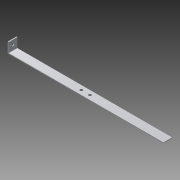
# Autodesk Inventor part: 爪２
Saved by Autodesk Inventor 2015 (Build 190159000, 159)
## iProperties
Created: 2015-05-17
Part Number: 爪２
Material: アルミニウム 6061
Document SubType Name: Modeling
Designer: Shun
Density: 2.7 g/cm^3
Appearance: アルミニウム - フラット
Mass: 5.09186 g
Surface Area: 42.039 cm^2
Volume: 1.88587 cm^3
Author: Shun
Autodesk Inventor part; units mm, degrees
ref_plane "YZ Plane" through (0, 0, 0) normal (1, 0, 0) x (0, 1, 0)
ref_plane "XZ Plane" through (0, 0, 0) normal (0, 1, 0) x (-1, 0, 0)
ref_plane "XY Plane" through (0, 0, 0) normal (0, 0, 1) x (1, 0, 0)
sketch "スケッチ1" plane through (0, 0, 0) normal (0, 0, 1) x (1, 0, 0)
  line L0 (-17.6, 4.0667) -> (162.4, 4.0667)
  line L1 (162.4, 4.0667) -> (162.4, -5.9333)
  line L2 (162.4, -5.9333) -> (-17.6, -5.9333)
  line L3 (-17.6, -5.9333) -> (-17.6, 4.0667)
  point P0 (0, 0)
  dimension "d0" = 10
  dimension "d1" = 180
  constraints: 8 end point, 2 parallel, 1 horizontal, 1 perpendicular
  measures "d0" distance of L2.end L0.start
  measures "d1" distance of L0.start L0.end
extrude "押し出し1" add sketch "スケッチ1" along normal blind 1
sketch "スケッチ3" plane through (0, 0, 1) normal (0, 0, 1) x (1, 0, 0)
  circle A0 centre (62.4, -0.9333) radius 1.5
  line L0 (-17.6, 4.0667) -> (-17.6, -5.9333) projected
  line L1 (-17.6, -5.9333) -> (162.4, -5.9333) projected
  line L2 (162.4, 4.0667) -> (-17.6, 4.0667) projected
  point P0 (0, 0)
  point P1 (72.4, -0.9333)
  dimension "d14" = 3
  dimension "d15" = 80
  dimension "d16" = 5
  dimension "d24" = 10
  dimension "d25" = 5
  constraints: 1 centre point
  measures "d14" diameter of A0
  measures "d15" distance from line of A0.centre L0
  measures "d16" distance from line of L1 A0.centre
  measures "d24" distance of point (72.4, -0.933) A0.centre
  measures "d25" distance from line of point (72.4, -0.933) L2
hole "穴2" at (62.4, -0.9333, 1) at (72.4, -0.9333, 1) direction (0, 0, -1) diameter 3.2 end through all
sketch "スケッチ4" plane through (0, 0, 1) normal (0, 0, 1) x (1, 0, 0)
  line L0 (-17.6, -5.9333) -> (162.4, -5.9333) projected
  line L1 (-17.6, 4.0667) -> (-16.6, 4.0667)
  line L2 (-16.6, 4.0667) -> (-16.6, -5.9333)
  line L3 (-16.6, -5.9333) -> (-17.6, -5.9333)
  line L4 (-17.6, -5.9333) -> (-17.6, 4.0667)
  point P0 (0, 0)
  dimension "d26" = 1
  constraints: 8 end point, 2 parallel, 1 horizontal, 1 perpendicular, 1 point on line
  measures "d26" distance of L2.end L3.end
extrude "押し出し2" add sketch "スケッチ4" along normal blind 11
sketch "スケッチ5" plane through (-16.6, -5.9333, 1) normal (1, 0, 0) x (0, 0, -1)
  line L0 (-11, 0) -> (-11, 10) projected
  line L1 (0, 0) -> (-11, 0) projected
  point P0 (1, 5.9333)
  point P1 (-6, 5)
  dimension "d29" = 5
  dimension "d30" = 5
  measures "d29" distance from line of point (-6, 5) L0
  measures "d30" distance from line of L1 point (-6, 5)
hole "穴3" at (-16.6, -0.9333, 7) direction (-1, 0, 0) diameter 3.2 end through all
